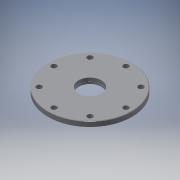
# Autodesk Inventor part: 零件7
Saved by Autodesk Inventor 2016 (Build 200138000, 138)
## iProperties
Created: 2016-12-22
Part Number: 零件7
Material: 一般
Document SubType Name: Modeling
Designer: Alex
Density: 1 g/cm^3
Appearance: 預設
Author: Alex
Autodesk Inventor part; units mm, degrees
ref_plane "YZ Plane" through (0, 0, 0) normal (1, 0, 0) x (0, 1, 0)
ref_plane "XZ Plane" through (0, 0, 0) normal (0, 1, 0) x (-1, 0, 0)
ref_plane "XY Plane" through (0, 0, 0) normal (0, 0, 1) x (1, 0, 0)
sketch "草圖1" plane through (0, 0, 0) normal (0, 0, 1) x (1, 0, 0)
  circle A0 centre (0, 0) radius 93.5
  dimension "d0" = 187
  constraints: 1 centre point, 1 coincident
  measures "d0" diameter of A0
extrude "擠出1" add sketch "草圖1" along normal blind 12
hole "孔1" at (0, 0, 12) direction (0, 0, -1) diameter 50 end through all counterbore diameter 50.8 counterbore depth 10
sketch "草圖2" plane through (0, 0, 12) normal (0, 0, 1) x (1, 0, 0)
  circle A0 centre (0, 0) radius 80 construction
  line L0 (0, 0) -> (56.5685, 56.5685) construction
  line L1 (0, 0) -> (80, 0) construction
  point P0 (0, 80)
  point P1 (-80, 0)
  point P2 (0, -80)
  point P3 (-56.5685, 56.5685)
  point P4 (-56.5685, -56.5685)
  point P5 (56.5685, -56.5685)
  dimension "d12" = 160
  dimension "d13" = 45
  constraints: 4 end point, 2 coincident, 1 equal length, 1 horizontal, 10 other
  measures "d13" angle of L1 L0
hole "孔2" at (0, 80, 12) at (-80, 0, 12) at (80, 0, 12) at (0, -80, 12) at (56.5685, 56.5685, 12) at (-56.5685, 56.5685, 12) at (-56.5685, -56.5685, 12) at (56.5685, -56.5685, 12) direction (0, 0, -1) diameter 12 end through all
chamfer "倒角1" distance 1 angle 45 2 edges at (-93.5, 0, 12) (-93.5, 0, 0)
